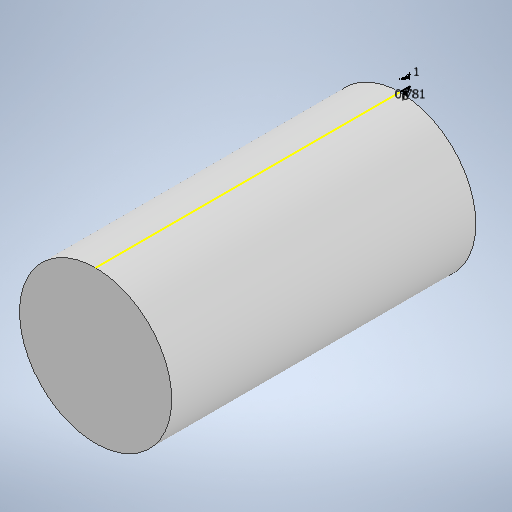
# Autodesk Inventor part: Peça9
Saved by Autodesk Inventor 2025.2 (Build 292293000, 293)
## iProperties
Created: 2025-03-25
Part Number: Peça9
Material: Genérico
Document SubType Name: Modeling
Designer: Formação
Density: 1 g/cm^3
Appearance: Padrão
Author: Formação
Autodesk Inventor part; units mm, degrees
ref_plane "YZ Plane" through (0, 0, 0) normal (1, 0, 0) x (0, 1, 0)
ref_plane "XZ Plane" through (0, 0, 0) normal (0, 1, 0) x (-1, 0, 0)
ref_plane "XY Plane" through (0, 0, 0) normal (0, 0, 1) x (1, 0, 0)
sketch "Esboço1" plane through (0, 0, 0) normal (0, 0, 1) x (1, 0, 0)
  circle A0 centre (0, 0) radius 7.5
  dimension "d0" = 15
  constraints: 2 coincident, 1 centre point
  measures "d0" diameter of A0
extrude "Extrusão1" add sketch "Esboço1" along normal mid plane 30
sketch "Esboço2" plane through (0, 0, 0) normal (1, 0, 0) x (0, 1, 0)
  line L0 (6.634, -15.5) -> (7.5, -15) construction
  line L1 (7.5, -15) -> (7.5, -16) construction
  line L2 (7.5, -16) -> (6.634, -15.5) construction
  line L3 (-7.5, -15) -> (7.5, -15) projected
  line L4 (7.5, -15) -> (7.5, -16)
  line L5 (7.5, -15) -> (7.5, 15) projected
  arc A0 (6.7617, -15.4262) -> (6.7617, -15.5738) centre (6.8043, -15.5) ccw
  line L6 (7.5, -16) -> (6.7617, -15.5738)
  line L7 (7.5, -15) -> (6.7617, -15.4262)
  point P0 (0, 0)
  point P1 (7.2113, -15.5)
  point P2 (6.7191, -15.5)
  dimension "d3" = 1
  dimension "d7" = 0.7809
  dimension "d8" = 0
  constraints: 12 end point, 5 point on line, 3 collinear, 3 point on circle, 3 tangent, 1 centre point, 7 other
  measures "d3" distance of L1.end L0.end
  measures "d7" horizontal distance of point (6.719, -15.5) L1.end
  measures "d8" vertical distance of A0.centre point (6.719, -15.5)
